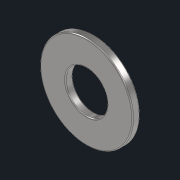
# Autodesk Inventor part: WSJ-STN-M5
Saved by Autodesk Inventor 2022 (Build 260153000, 153)
## iProperties
Created: 2021-02-03
Part Number: WSJ-STN-M5
Material: 鋼、炭素鋼
Document SubType Name: Modeling
Designer: Yuta Kage
Mass: 0.025625 g
Surface Area: 1.22145 cm^2
Volume: 0.0241746 cm^3
Density: 7.85 g/cm^3
Appearance: 半つや出し
Description: 3Dプリント
購入先: ミスミ
在庫数: 0.0
Author: Yuta Kage
Autodesk Inventor part; units mm, degrees
ref_plane "YZ Plane" through (0, 0, 0) normal (1, 0, 0) x (0, 1, 0)
ref_plane "XZ Plane" through (0, 0, 0) normal (0, 1, 0) x (-1, 0, 0)
ref_plane "XY Plane" through (0, 0, 0) normal (0, 0, 1) x (1, 0, 0)
sketch "スケッチ1" plane through (0, 0, 0) normal (0, 0, 1) x (1, 0, 0)
  circle A0 centre (0, 0) radius 2.25
  circle A1 centre (0, 0) radius 5
  dimension "d0" = 4.5
  dimension "d1" = 10
  constraints: 2 centre point, 2 coincident
  measures "d0" diameter of A0
  measures "d1" diameter of A1
extrude "押し出し1" add sketch "スケッチ1" along normal blind 0.8
fillet "フィレット1" radius 0.1 4 edges at (-5, 0, 0.8) (-5, 0, 0) (-2.25, 0, 0.8) (-2.25, 0, 0)
